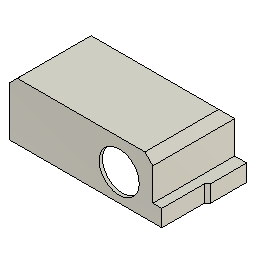
1_Assembly Camera v20 (Autodesk Fusion 360 archive; units mm, degrees)
design "Camera"
Autodesk Fusion 360 part; units mm, degrees
sketch "Cam" plane through (0, 0, 0) normal (0, 0, 1) x (1, 0, 0)
  line L0 (-62.75, 35.75) -> (62.75, 35.75)
  line L1 (62.75, 35.75) -> (62.75, -35.75)
  line L2 (62.75, -35.75) -> (-62.75, -35.75)
  line L3 (-62.75, -35.75) -> (-62.75, 35.75)
  line L4 (62.75, -35.75) -> (70.55, -35.75)
  line L5 (70.55, -35.75) -> (70.55, 1.75)
  line L6 (70.55, 1.75) -> (73.25, 4.45)
  line L7 (73.25, 4.45) -> (73.25, 35.75)
  line L8 (73.25, 35.75) -> (62.75, 35.75)
  line L9 (-62.75, 35.75) -> (62.75, -35.75) construction
  line L10 (-62.75, -35.75) -> (62.75, 35.75) construction
  dimension "d122" = 125.5
  dimension "d123" = 71.5
  dimension "d126" = 10.5
  dimension "d127" = 7.8
  dimension "d395" = 135
  dimension "d396" = 31.3
  constraint horizontal L0
  constraint vertical L1
  constraint horizontal L2
  constraint vertical L3
  constraint perpendicular L1 L4
  constraint perpendicular L4 L5
  constraint perpendicular L4 L7
  constraint perpendicular L7 L8
  constraint coincident origin L10
  constraint coincident origin L9
  measures "d122" distance of L0.start L0.end
  measures "d123" distance of L0.start L2.end
  measures "d126" distance of L0.end L7.end
  measures "d127" distance of L1.end L4.end
  measures "d395" angle of L5 L6
  measures "d396" distance of L6.end L7.end
extrude "Extrude2" add sketch "Cam" along normal blind 50 contours L0 L1 L2 L3
chamfer "Chamfer2" distance 7 angle 45 3 edges at (-62.75, 0, 50) (0, 35.75, 50) (62.75, 0, 50)
shell "Shell1" thickness 3 removed faces 1 at (20.9167, -11.9167, 0)
extrude "Extrude3" add sketch "Cam" along normal blind 14.7 contours L1 L4 L5 L6 L7 L8
sketch "Cam hole" plane through (0, -35.75, 0) normal (0, -1, 0) x (1, 0, 0)
  line L0 (62.75, 43) -> (55.75, 50)
  line L1 (55.75, 50) -> (-55.75, 50)
  line L2 (-55.75, 50) -> (-62.75, 43)
  line L3 (-62.75, 43) -> (-62.75, 0)
  line L4 (-62.75, 0) -> (70.55, 0)
  line L5 (70.55, 0) -> (70.55, 14.7)
  line L6 (70.55, 14.7) -> (62.75, 14.7)
  line L7 (62.75, 14.7) -> (62.75, 43)
  circle A0 centre (33.25, 23.5) radius 17.5
  dimension "d137" = 35
  dimension "d154" = 23.5
  dimension "d155" = 29.5
  measures "d137" diameter of A0
  measures "d154" distance of L4 A0.centre
  measures "d155" distance of L7 A0.centre
extrude "Extrude4" cut sketch "Cam hole" against normal blind 20 contours A0
sketch "Cam Fix" plane through (0, 0, 0) normal (0, 0, -1) x (1, 0, 0)
  line L0 (-59.75, -32.75) -> (-59.75, 32.75)
  line L1 (-59.75, 32.75) -> (59.75, 32.75)
  line L2 (59.75, 32.75) -> (59.75, -32.75)
  line L3 (59.75, -32.75) -> (-59.75, -32.75)
  line L4 (70.55, 35.75) -> (-62.75, 35.75)
  line L5 (-62.75, 35.75) -> (-62.75, -35.75)
  line L6 (-62.75, -35.75) -> (73.25, -35.75)
  line L7 (73.25, -35.75) -> (73.25, -4.45)
  line L8 (73.25, -4.45) -> (70.55, -1.75)
  line L9 (70.55, -1.75) -> (70.55, 35.75)
  line L10 (-59.75, 32.75) -> (-49.75, 32.75)
  line L11 (-49.75, 32.75) -> (-49.75, 22.75)
  line L12 (-49.75, 22.75) -> (-59.75, 22.75)
  line L13 (-59.75, 22.75) -> (-59.75, 32.75)
  line L14 (-59.75, -32.75) -> (-49.75, -32.75)
  line L15 (-49.75, -32.75) -> (-49.75, -22.75)
  line L16 (-49.75, -22.75) -> (-59.75, -22.75)
  line L17 (-59.75, -22.75) -> (-59.75, -32.75)
  line L18 (-59.75, 32.75) -> (-49.75, 22.75) construction
  line L19 (-59.75, -22.75) -> (-49.75, -32.75) construction
  circle A0 centre (-54.75, 27.75) radius 2.6
  circle A1 centre (64.75, 27.75) radius 2.6
  circle A2 centre (64.75, -27.75) radius 2.6
  circle A3 centre (-54.75, -27.75) radius 2.6
  line L20 (59.75, 32.75) -> (69.75, 32.75)
  line L21 (69.75, 32.75) -> (69.75, 22.75)
  line L22 (69.75, 22.75) -> (59.75, 22.75)
  line L23 (59.75, 22.75) -> (59.75, 32.75)
  line L24 (59.75, -22.75) -> (69.75, -22.75)
  line L25 (69.75, -22.75) -> (69.75, -32.75)
  line L26 (69.75, -32.75) -> (59.75, -32.75)
  line L27 (59.75, -32.75) -> (59.75, -22.75)
  line L28 (59.75, -22.75) -> (69.75, -32.75) construction
  line L29 (59.75, 32.75) -> (69.75, 22.75) construction
  dimension "d140" = 10
  dimension "d141" = 10
  dimension "d142" = 10
  dimension "d143" = 10
  dimension "d148" = 5.2
  dimension "d149" = 5.2
  dimension "d150" = 5.2
  dimension "d151" = 5.2
  dimension "d156" = 10
  dimension "d157" = 10
  dimension "d158" = 10
  dimension "d159" = 10
  constraint horizontal L10
  constraint vertical L11
  constraint horizontal L12
  constraint vertical L13
  constraint coincident L0.end L1.start
  constraint horizontal L14
  constraint vertical L15
  constraint horizontal L16
  constraint vertical L17
  constraint coincident L0.start L3.end
  constraint coincident L1.end L2.start
  constraint midpoint L18 A0.centre
  constraint midpoint L19 A3.centre
  constraint horizontal L20
  constraint vertical L21
  constraint horizontal L22
  constraint vertical L23
  constraint horizontal L24
  constraint vertical L25
  constraint horizontal L26
  constraint vertical L27
  constraint midpoint A1.centre L29
  constraint midpoint A2.centre L28
  constraint coincident L2.end L3.start
  measures "d140" distance of L0.end L10.end
  measures "d141" distance of L0.end L12.end
  measures "d142" distance of L0.start L14.end
  measures "d143" distance of L0.start L16.end
  measures "d148" diameter of A0
  measures "d149" diameter of A1
  measures "d150" diameter of A2
  measures "d151" diameter of A3
  measures "d156" distance of L1.end L20.end
  measures "d157" distance of L1.end L22.end
  measures "d158" distance of L24.start L24.end
  measures "d159" distance of L2.end L24.start
extrude "Extrude5" add sketch "Cam Fix" against normal blind 10 contours L0 L3 L14 L15 L16 L17 | L0 L1 L10 L11 L12 L13 | A0 | A3
extrude "Extrude6" cut sketch "Cam Fix" against normal blind 3.1 contours A0 | A1 | A2 | A3
equation "Trous_Vis_diam2 = 2.2 mm"
equation "d175 = Trous_Vis_diam2"
equation "d176 = Trous_Vis_diam2"
equation "d179 = Trous_Vis_diam2"
equation "d180 = Trous_Vis_diam2"
equation "d183 = Trous_Vis_diam2"
equation "d185 = Trous_Vis_diam2"
equation "d186 = Trous_Vis_diam2"
equation "d187 = Trous_Vis_diam2"
equation "d198 = Trous_Vis_diam2"
equation "d199 = Trous_Vis_diam2"
equation "d200 = Trous_Vis_diam2"
equation "d201 = Trous_Vis_diam2"
equation "d365 = Trous_Vis_diam2"
equation "d367 = Trous_Vis_diam2"
equation "d368 = Trous_Vis_diam2"
equation "d369 = Trous_Vis_diam2"
named bodies: "Cam"

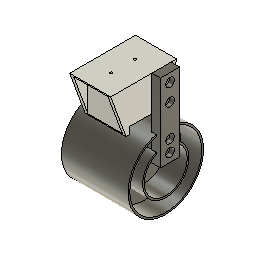
design "Under Camera"
Autodesk Fusion 360 part; units mm, degrees
sketch "Sketch1" plane through (0, -227.1998, 566.5) normal (1, 0, 0) x (0, 1, 0) in component "Under Cam"
  line L0 (-26, -3.5) -> (12.5005, -3.5)
  line L1 (12.5005, -3.5) -> (8.0001, -24)
  line L2 (8.0001, -24) -> (-15.3, -24)
  line L3 (-15.3, -24) -> (-15.3, -28.1777)
  line L4 (-15.3, -28.1777) -> (-17, -28.1777)
  line L5 (-17, -28.1777) -> (-26, -3.5)
  line L6 (3.7005, -3.5) -> (3.7005, -24) construction
  circle A0 centre (3.7005, -8.5) radius 0.75
  circle A1 centre (3.7005, -18.5) radius 0.75
  dimension "d282" = 8.8
  dimension "d283" = 1.5
  dimension "d284" = 5
  dimension "d285" = 1.5
  dimension "d286" = 10
  constraint horizontal L0
  constraint parallel L0 L2
  constraint perpendicular L2 L3
  constraint perpendicular L3 L4
  constraint coincident L0 L6.start
  constraint coincident L2 L6.end
  constraint perpendicular L2 L6
  constraint coincident L6 A0.centre
  constraint coincident L6 A1.centre
  measures "d282" distance of L0.end L6.start
  measures "d283" diameter of A0
  measures "d284" distance of L0 A0.centre
  measures "d285" diameter of A1
  measures "d286" distance of A0.centre A1.centre
extrude "Extrude1" add sketch "Sketch1" against normal blind 24 contours L0 L1 L2 L3 L4 L5 | A0 | A1 makes body 1 in component "Under Cam"
ref_plane "WorkPlane2" through (-12, -257.4998, 540.4111) normal (0, 1, 0) x (0, 0, -1) in component "Under Cam"
sketch "Sketch2" plane through (-71.456, -257.4998, 540.4111) normal (0, 1, 0) x (1, 0, 0) in component "Under Cam"
  line L0 (71.456, 2.0889) -> (71.456, -22.5888)
  line L1 (71.456, -22.5888) -> (47.456, -22.5888)
  line L2 (47.456, -22.5888) -> (47.456, 2.0889)
  line L3 (47.456, 2.0889) -> (71.456, 2.0889)
  line L4 (49.456, -21.5888) -> (69.456, -21.5888)
  line L5 (69.456, -21.5888) -> (69.456, 2.0889)
  line L6 (69.456, 2.0889) -> (49.456, 2.0889)
  line L7 (49.456, 2.0889) -> (49.456, -21.5888)
  dimension "d273" = 2
  dimension "d274" = 2
  dimension "d275" = 1
  constraint horizontal L4
  constraint vertical L5
  constraint horizontal L6
  constraint vertical L7
  constraint coincident L3 L5.end
  measures "d273" horizontal distance of L1.end L4.start
  measures "d274" horizontal distance of L0.end L4.end
  measures "d275" vertical distance of L0.end L4.end
extrude "Extrude2" cut sketch "Sketch2" along normal blind 13 contours L3 L4 L5 L6 L7 bodies 1 in component "Under Cam"
extrude "Extrude4" cut sketch "Sketch1" against normal blind 10 contours A0 | A1 bodies 1 in component "Under Cam"
sketch "Sketch3" plane through (0, -227.1998, 566.5) normal (1, 0, 0) x (0, 1, 0) in component "Under Cam"
  line L0 (-1.8995, -3.5) -> (9.3005, -3.5)
  line L1 (9.3005, -3.5) -> (9.3005, -49)
  line L2 (9.3005, -49) -> (-1.8995, -49)
  line L3 (-1.8995, -49) -> (-1.8995, -3.5)
  line L4 (-26, -3.5) -> (12.5005, -3.5)
  line L5 (-26, -3.5) -> (12.5005, -3.5) construction
  line L6 (3.7005, -3.5) -> (3.7005, -49) construction
  circle A0 centre (3.7005, -8.5) radius 1.1
  circle A1 centre (3.7005, -18.5) radius 1.1
  line L7 (3.7005, -49) -> (3.7005, -77.9127) construction
  point P0 (3.7005, -8.5)
  point P1 (3.7005, -18.5)
  dimension "d278" = 11.2
  dimension "d281" = 8.8
  dimension "d289" = 2.2
  dimension "d290" = 2.2
  constraint horizontal L0
  constraint vertical L1
  constraint horizontal L2
  constraint vertical L3
  constraint coincident L4.start L5.start
  constraint coincident L4.end L5.end
  constraint coincident L0.end L5
  constraint midpoint L0 L6.start
  constraint perpendicular L0 L6
  constraint coincident P0 A0.centre
  constraint coincident P1 A1.centre
  constraint perpendicular L2 L7
  measures "d278" distance of L0.start L0.end
  measures "d281" distance of L4.end L6.start
  measures "d289" diameter of A0
  measures "d290" diameter of A1
extrude "Extrude3" add sketch "Sketch3" along normal blind 5 separate body makes body 2 in component "Under Cam"
sketch "Sketch4" plane through (5, 0, 0) normal (1, 0, 0) x (0, 1, 0) in component "Under Cam"
  circle A0 centre (-223.4993, 548) radius 1.1
  circle A1 centre (-223.4993, 558) radius 1.1
  line L0 (-229.0993, 517.5) -> (-217.8993, 517.5)
  line L1 (-217.8993, 517.5) -> (-217.8993, 563)
  line L2 (-217.8993, 563) -> (-229.0993, 563)
  line L3 (-229.0993, 563) -> (-229.0993, 517.5)
  circle A2 centre (-223.4993, 558) radius 2.5
  circle A3 centre (-223.4993, 548) radius 2.5
  line L4 (-223.4993, 548) -> (-223.4993, 517.5) construction
  dimension "d291" = 5
  dimension "d292" = 5
  constraint concentric A1 A2
  constraint concentric A0 A3
  constraint coincident A0.centre A3.centre
  constraint midpoint L0 L4.end
  measures "d291" diameter of A2
  measures "d292" diameter of A3
sketch "Sketch6" plane through (0, -227.1998, 566.5) normal (1, 0, 0) x (0, 1, 0) in component "Under Cam"
  line L0 (-1.8995, -49) -> (9.3005, -49)
  line L1 (3.7005, -49) -> (3.7005, -32.5726) construction
  circle A0 centre (3.7005, -54.5726) radius 22
  circle A1 centre (3.7005, -54.5726) radius 21
  circle A2 centre (3.7005, -54.5726) radius 13.5
  circle A3 centre (3.7005, -54.5726) radius 12.5
  line L2 (9.3005, -49) -> (9.3005, -33.2972)
  line L3 (-1.8995, -49) -> (-1.8995, -33.2972)
  circle A4 centre (3.7005, -37) radius 0.75
  circle A5 centre (3.7005, -44) radius 0.75
  point P0 (9.3005, -49)
  point P1 (-1.8995, -49)
  dimension "d295" = 44
  dimension "d298" = -1
  dimension "d299" = -8.5
  dimension "d300" = -9.5
  dimension "d305" = 1.5
  dimension "d306" = 1.5
  dimension "d307" = 5
  dimension "d308" = 7
  constraint coincident P1 L0.start
  constraint coincident P0 L0.end
  constraint midpoint L0 L1.start
  constraint perpendicular L0 L1
  constraint coincident L1 A0.centre
  constraint coincident A0 L2.end
  constraint vertical L2
  constraint coincident A0 L3.end
  constraint perpendicular L0 L3
  constraint coincident L1.end A0
  constraint coincident L1 A4.centre
  constraint coincident L1 A5.centre
  measures "d295" diameter of A0
  measures "d305" diameter of A4
  measures "d306" diameter of A5
  measures "d307" distance of L1.start A5.centre
  measures "d308" distance of A4.centre A5.centre
extrude "Extrude6" add sketch "Sketch6" against normal blind 36.5 separate body contours L0 A3 L2 L3 | L0 A3 L2 L3 | A2 A3 L2 L3 | A2 A3 L2 L3 | A1 A2 L2 L3 | A1 A2 L2 L3 | A0 A1 L2 L3 | A0 A1 L2 L3 | A4 | A5 makes body 3 in component "Under Cam"
extrude "Extrude7" cut sketch "Sketch6" against normal blind 10 contours L0 A3 L2 L3 | A1 A2 L2 L3 picked at (3.532, -55.0208) picked at (-4.7622, -38.1727) bodies 3 in component "Under Cam"
extrude "Extrude8" add sketch "Sketch6" along normal blind 2.5 contours A2 A3 L2 L3 | A0 A1 L2 L3 picked at (-3.0056, -43.6595) picked at (-3.9032, -34.6912) bodies 3 in component "Under Cam"
extrude "Extrude9" cut sketch "Sketch6" against normal blind 10 contours A4 | A5 bodies 3 in component "Under Cam"
sketch "Sketch7" plane through (5, 0, 0) normal (1, 0, 0) x (0, 1, 0) in component "Under Cam"
  line L0 (-229.0993, 517.5) -> (-217.8993, 517.5)
  line L1 (-217.8993, 517.5) -> (-217.8993, 563)
  line L2 (-217.8993, 563) -> (-229.0993, 563)
  line L3 (-229.0993, 563) -> (-229.0993, 517.5)
  circle A0 centre (-223.4993, 529.5) radius 1.1
  circle A1 centre (-223.4993, 522.5) radius 1.1
  circle A2 centre (-223.4993, 529.5) radius 2.5
  circle A3 centre (-223.4993, 522.5) radius 2.5
  circle A4 centre (-223.4993, 558) radius 1.1
  circle A5 centre (-223.4993, 548) radius 1.1
  point P0 (-223.4993, 529.5)
  point P1 (-223.4993, 522.5)
  dimension "d311" = 2.2
  dimension "d312" = 2.2
  dimension "d313" = 5
  dimension "d314" = 5
  constraint coincident P0 A0.centre
  constraint coincident P1 A1.centre
  constraint concentric A0 A2
  constraint concentric A1 A3
  measures "d311" diameter of A0
  measures "d312" diameter of A1
  measures "d313" diameter of A2
  measures "d314" diameter of A3
extrude "Extrude5" cut sketch "Sketch4" sketch "Sketch7" against normal blind 2.5 contours A2 | A3 of sketch 2 contours A2 | A3 bodies 2 in component "Under Cam"
extrude "Extrude10" cut sketch "Sketch7" against normal blind 5 contours A0 | A1 bodies 2 in component "Under Cam"
sketch "Sketch8" plane through (0, 0, 563) normal (0, 0, 1) x (-1, 0, 0) in component "Under Cam"
  line L0 (0, 253.1998) -> (0, 214.6993)
  line L1 (0, 214.6993) -> (24, 214.6993)
  line L2 (24, 214.6993) -> (24, 253.1998)
  line L3 (24, 253.1998) -> (0, 253.1998)
  line L4 (12, 214.6993) -> (12, 253.1998) construction
  circle A0 centre (12, 226.9495) radius 0.75
  circle A1 centre (12, 240.9495) radius 0.75
  line L5 (12, 233.9495) -> (0, 233.9495) construction
  dimension "d389" = 1.5
  dimension "d390" = 1.5
  dimension "d391" = 7
  dimension "d392" = 7
  constraint midpoint L1 L4.start
  constraint midpoint L3 L4.end
  constraint coincident L4 A0.centre
  constraint coincident L4 A1.centre
  constraint midpoint L4 L5.start
  constraint midpoint L0 L5.end
  measures "d389" diameter of A0
  measures "d390" diameter of A1
  measures "d391" distance of A1.centre L5.start
  measures "d392" distance of A0.centre L5.start
extrude "Extrude11" cut sketch "Sketch8" against normal blind 10 contours A0 | A1 bodies 1 in component "Under Cam"
component "Under Cam" placed x (1, 0, 0) y (0, 1, 0) z (0, 0, 1) at (0, 0, 0)
equation "Trous_Vis_diam2 = 2.2 mm"
equation "d175 = Trous_Vis_diam2"
equation "d176 = Trous_Vis_diam2"
equation "d179 = Trous_Vis_diam2"
equation "d180 = Trous_Vis_diam2"
equation "d183 = Trous_Vis_diam2"
equation "d185 = Trous_Vis_diam2"
equation "d186 = Trous_Vis_diam2"
equation "d187 = Trous_Vis_diam2"
equation "d198 = Trous_Vis_diam2"
equation "d199 = Trous_Vis_diam2"
equation "d200 = Trous_Vis_diam2"
equation "d201 = Trous_Vis_diam2"
equation "d365 = Trous_Vis_diam2"
equation "d367 = Trous_Vis_diam2"
equation "d368 = Trous_Vis_diam2"
equation "d369 = Trous_Vis_diam2"
named bodies: "support double cam", "fixation latérale", "Cylindre"

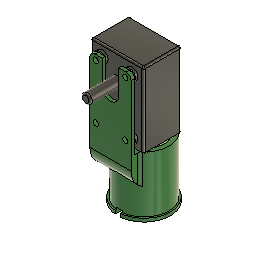
design "Support motor rotor"
Autodesk Fusion 360 part; units mm, degrees
sketch "Sketch1" plane through (0, 0, 0) normal (0, 0, 1) x (1, 0, 0)
  circle A0 centre (0, 0) radius 12.4
  circle A1 centre (0, 0) radius 13.4
  circle A2 centre (0, 0) radius 1.1
  circle A3 centre (0, 0) radius 15
  circle A4 centre (0, 0) radius 16
  dimension "d1" = 24.8
  dimension "d2" = 1
  dimension "d8" = 2.2
  dimension "d103" = 30
  dimension "d117" = 32
  constraint coincident A0.centre A1.centre
  constraint concentric A0 A2
  measures "d1" diameter of A0
  measures "d8" diameter of A2
  measures "d103" diameter of A3
  measures "d117" diameter of A4
extrude "Extrude1" add sketch "Sketch1" against normal blind 2 contours A0 | A1 | A3 makes body 1
extrude "Extrude2" add sketch "Sketch1" along normal blind 34 contours A1 bodies 1
ref_plane "WorkPlane2" through (0, -15, 0) normal (0, 1, 0) x (0, 0, 1)
sketch "Sketch3" plane through (0, -15, 0) normal (0, 1, 0) x (1, 0, 0)
sketch "Sketch4" plane through (0, -15, 0) normal (0, 1, 0) x (1, 0, 0)
  line L0 (-13.4, -34) -> (13.4, -34)
  line L1 (-8.4, -34) -> (-3.3, -34)
  line L2 (7.8, -34) -> (7.8, -14)
  line L3 (7.8, -14) -> (-8.4, -14)
  line L4 (-8.4, -14) -> (-8.4, -34)
  line L5 (9.2, -77) -> (9.2, -34)
  line L6 (9.2, -34) -> (-15.8, -34)
  line L7 (-15.8, -34) -> (-15.8, -77)
  line L8 (-3.3, -77) -> (-3.3, -34) construction
  line L9 (-8.3, -77) -> (-8.3, -62.0106)
  line L10 (1.7, -77) -> (1.7, -62.0106)
  line L11 (-15.8, -77) -> (-8.3, -77)
  line L12 (1.7, -77) -> (9.2, -77)
  arc A0 (1.7, -62.0106) -> (-8.3, -62.0106) centre (-3.3, -62.0106) ccw
  line L13 (-12.3, -74) -> (5.7, -74) construction
  line L14 (5.7, -74) -> (5.7, -41) construction
  line L15 (5.7, -41) -> (-12.3, -41) construction
  line L16 (-12.3, -41) -> (-12.3, -74) construction
  circle A1 centre (5.7, -41) radius 1.6
  circle A2 centre (-12.3, -41) radius 1.6
  circle A3 centre (-12.3, -74) radius 1.6
  circle A4 centre (5.7, -74) radius 1.6
  line L17 (13.4, 0) -> (-13.4, 0)
  line L18 (9.2, -34) -> (-15.8, -34)
  line L19 (-15.8, -34) -> (-15.8, -14)
  line L20 (-15.8, -14) -> (9.2, -14)
  line L21 (9.2, -14) -> (9.2, -34)
  dimension "d55" = 5
  dimension "d57" = 25
  dimension "d58" = 43
  dimension "d62" = 7.4
  dimension "d64" = 10
  dimension "d66" = 33
  dimension "d67" = 18
  dimension "d69" = 3.5
  dimension "d70" = 3.5
  dimension "d71" = 3.2
  dimension "d72" = 3.2
  dimension "d73" = 3.2
  dimension "d74" = 3.2
  dimension "d76" = 7
  dimension "d85" = 20
  constraint horizontal L1
  constraint vertical L2
  constraint horizontal L3
  constraint vertical L4
  constraint coincident L0 L1.start
  constraint horizontal L11
  constraint vertical L5
  constraint horizontal L6
  constraint vertical L7
  constraint coincident L1.start L6
  constraint midpoint L6 L1.end
  constraint coincident L8 A0.centre
  constraint tangent L9 A0
  constraint perpendicular L9 L11
  constraint coincident L10.start L11
  constraint tangent L10 A0
  constraint perpendicular L10 L11
  constraint collinear L11 L12
  constraint coincident L8.start L11
  constraint horizontal L13
  constraint vertical L14
  constraint horizontal L15
  constraint vertical L16
  constraint coincident L14.end L15.start
  constraint coincident L15.end L16.start
  constraint coincident L13.start L16.end
  constraint coincident L13.end L14.start
  constraint horizontal L18
  constraint vertical L19
  constraint horizontal L20
  constraint vertical L21
  constraint coincident L6.end L7.start
  measures "d55" distance of L0.start L1.start
  measures "d57" distance of L7.end L5.start
  measures "d58" distance of L7.end L6.end
  measures "d62" distance of L1.start L6.end
  measures "d64" diameter of A0
  measures "d66" distance of L13.start L15.end
  measures "d67" distance of L13.start L13.end
  measures "d69" distance of L5 L14.end
  measures "d70" distance of L7 L15.end
  measures "d71" diameter of A1
  measures "d72" diameter of A2
  measures "d73" diameter of A3
  measures "d74" diameter of A4
  measures "d76" distance of L1 L14.end
  measures "d85" distance of L2.start L2.end
extrude "Extrude6" add sketch "Sketch4" against normal blind 2 separate body makes body 2
extrude "Extrude7" add sketch "Sketch4" along normal blind 13 contours L0 L4 L6 L18 L19 L20 | L0 L1 L2 L3 L4 L6 L18 L20 | L0 L2 L6 L18 L20 L21 bodies 1 2
extrude "Extrude9" cut 1 faces at (8.5831, -0.6707, 0) along direction (0, 0, 1) blind 35 on bodies 1 bodies 1
extrude "Extrude10" add 1 faces at (14.4108, -0.7452, 0) along direction (0, 0, 1) blind 34 on bodies 1 bodies 1
fillet "Fillet3" radius 3 2 edges at (9.2, -16, 77) (-15.8, -16, 77) on bodies 1
fillet "Fillet2" radius 12.5 1 edges at (-3.3, -17, 14) on bodies 1
fillet "Fillet6" radius 2.5 1 edges at (9.2, -11.8474, 25.1937) on bodies 1
extrude "Extrude13" add sketch "Sketch1" against normal blind 2 contours A4 bodies 1
sketch "Sketch6" plane through (0, 0, -2) normal (0, 0, -1) x (1, 0, 0)
  line L0 (1.6, -16.8286) -> (-1.6, -16.8286)
  line L1 (-1.6, -16.8286) -> (-1.6, 16.8286)
  line L2 (-1.6, 16.8286) -> (1.6, 16.8286)
  line L3 (1.6, 16.8286) -> (1.6, -16.8286)
  line L4 (1.6, -16.8286) -> (-1.6, 16.8286) construction
  line L5 (-1.6, -16.8286) -> (1.6, 16.8286) construction
  circle A0 centre (0, 0) radius 7.5
  circle A1 centre (0, 0) radius 1.1
  circle A2 centre (0, 0) radius 16
  dimension "d108" = 3.2
  dimension "d111" = 15
  constraint perpendicular L0 L1
  constraint parallel L0 L2
  constraint parallel L1 L3
  constraint horizontal L0
  constraint coincident L4 A0.centre
  constraint coincident L5 A0.centre
  constraint coincident A0.centre A1.centre
  measures "d108" distance of L1.end L2.end
  measures "d111" diameter of A0
extrude "Extrude11" cut sketch "Sketch6" against normal blind 3 contours L1 L3 A0 A2 | L1 L3 A0 A2 bodies 1
fillet "Fillet7" radius 5 1 edges at (-15.8, -2, 24) on bodies 1
sketch "Sketch7" plane through (0, 0, -2) normal (0, 0, -1) x (1, 0, 0)
  circle A0 centre (0, 0) radius 12.4
  line L0 (0, 0) -> (0, -12.4) construction
  line L1 (-10.745, 10.3072) -> (-12.3181, 8.3641)
  arc A1 (-12.3181, 8.3641) -> (-8.802, 8.7342) centre (-10.375, 6.7911) ccw
  arc A2 (-10.375, 6.7911) -> (-10.745, 10.3072) centre (-8.802, 8.7342) ccw
  dimension "d115" = 5
  dimension "d116" = 5
  constraint coincident A0.centre L0.start
  constraint coincident A0 L0.end
  constraint vertical L0
  constraint coincident A0 A1.centre
  constraint coincident A0 A1.end
  constraint tangent L1 A1
  measures "d115" diameter of A1
  measures "d116" diameter of A2
extrude "Extrude12" cut sketch "Sketch7" against normal through all contours A0 L1 A1 A2 bodies 1
copy_body "Body->Comp2" bodies 1 removing the originals makes body 3 in component "Support Motor"
sketch "Sketch1 (2)" plane through (0, 0, 0) normal (0, 0, 1) x (1, 0, 0) in component "Head Motor v3"
  line L0 (-16, -23) -> (16, -23)
  line L1 (16, -23) -> (16, 23)
  line L2 (16, 23) -> (-16, 23)
  line L3 (-16, 23) -> (-16, -23)
  line L4 (-16, -23) -> (16, 23) construction
  line L5 (16, -23) -> (-16, 23) construction
  dimension "d1_1" = 46
  dimension "d2_1" = 32
  constraint perpendicular L0 L1
  constraint parallel L0 L2
  constraint parallel L1 L3
  constraint horizontal L0
  constraint coincident L4 origin
  constraint coincident L5 origin
  measures "d1_1" distance of L0.end L1.end
  measures "d2_1" distance of L1.end L2.end
extrude "Extrude1'" add sketch "Sketch1 (2)" along normal blind 23 separate body makes body 4 in component "Head Motor v3"
sketch "Sketch2" plane through (0, 0, 23) normal (0, 0, 1) x (-1, 0, 0) in component "Head Motor v3"
  line L0 (16, -23) -> (16, 23)
  line L1 (16, 23) -> (-16, 23)
  line L2 (-16, 23) -> (-16, -23)
  line L3 (-16, -23) -> (16, -23)
  line L4 (-9, 16.5) -> (9, 16.5) construction
  line L5 (9, 16.5) -> (9, -16.5) construction
  line L6 (9, -16.5) -> (-9, -16.5) construction
  line L7 (-9, -16.5) -> (-9, 16.5) construction
  line L8 (-9, 16.5) -> (9, -16.5) construction
  line L9 (9, 16.5) -> (-9, -16.5) construction
  circle A0 centre (-9, -16.5) radius 3.5
  circle A1 centre (9, -16.5) radius 3.5
  circle A2 centre (-9, 16.5) radius 3.5
  circle A3 centre (9, 16.5) radius 3.5
  line L10 (0, -23) -> (0, 23) construction
  circle A4 centre (0, -8) radius 3
  circle A5 centre (9, -16.5) radius 1.5
  circle A6 centre (-9, -16.5) radius 1.5
  circle A7 centre (9, 16.5) radius 1.5
  circle A8 centre (-9, 16.5) radius 1.5
  dimension "d5_1" = 33
  dimension "d6_1" = 18
  dimension "d7" = 7
  dimension "d8_1" = 7
  dimension "d9" = 7
  dimension "d10" = 7
  dimension "d13" = 6
  dimension "d14" = 15
  dimension "d34" = 3
  dimension "d35" = 3
  dimension "d36" = 3
  dimension "d37" = 3
  constraint perpendicular L4 L5
  constraint parallel L4 L6
  constraint parallel L5 L7
  constraint horizontal L4
  constraint coincident L8 origin
  constraint coincident L9 origin
  constraint coincident L6.end L7.start
  constraint coincident L5.end L6.start
  constraint coincident L4.start L7.end
  constraint coincident L4.end L5.start
  constraint midpoint L3 L10.start
  constraint midpoint L1 L10.end
  constraint coincident L10 A4.centre
  constraint concentric A1 A5
  constraint concentric A3 A7
  constraint concentric A2 A8
  measures "d5_1" distance of L4.end L5.end
  measures "d6_1" distance of L5.end L6.end
  measures "d7" diameter of A0
  measures "d8_1" diameter of A1
  measures "d9" diameter of A2
  measures "d10" diameter of A3
  measures "d13" diameter of A4
  measures "d14" distance of L3 A4.centre
  measures "d34" diameter of A5
  measures "d35" diameter of A6
  measures "d36" diameter of A7
  measures "d37" diameter of A8
extrude "Extrude2'" add sketch "Sketch2" along normal blind 2 contours A0 | A1 | A2 | A3 bodies 4 in component "Head Motor v3"
extrude "Extrude3" add sketch "Sketch2" along normal blind 19 contours A4 bodies 4 in component "Head Motor v3"
fillet "Fillet1" radius 1 4 faces at (16, -7.6667, 7.6667) (-5.3333, -23, 7.6667) (-16, 7.6667, 7.6667) (5.3333, 23, 7.6667) on bodies 4 in component "Head Motor v3"
fillet "Fillet2'" radius 0.5 1 edges at (-5.7369, -15.2343, 25) 4 faces at (6.1853, 16.7484, 25) (6.1853, -16.2516, 25) (-11.8147, 16.7484, 25) (-11.8147, -16.2516, 25) on bodies 4 in component "Head Motor v3"
fillet "Fillet3'" radius 1 1 faces at (0.5, 8.866, 42) on bodies 4 in component "Head Motor v3"
sketch "Sketch4 (2)" plane through (-3, 23, 11.5) normal (0, 1, 0) x (-1, 0, 0) in component "Head Motor v3"
sketch "Sketch5" plane through (0, -23, 0) normal (0, -1, 0) x (1, 0, 0) in component "Head Motor v3"
  line L0 (-15, 1) -> (15, 1)
  line L1 (15, 1) -> (15, 22)
  line L2 (15, 22) -> (-15, 22)
  line L3 (-15, 22) -> (-15, 1)
  circle A0 centre (3, 10) radius 12
  point P0 (16, 22)
  dimension "d25" = 24
  dimension "d26" = 10
  dimension "d27" = 13
  measures "d25" diameter of A0
  measures "d26" vertical distance of origin A0.centre
  measures "d27" horizontal distance of A0.centre P0
extrude "Extrude5" add sketch "Sketch5" along normal blind 31 contours L0 A0 | L0 A0 bodies 4 in component "Head Motor v3"
sketch "Sketch8" plane through (0, -54, 0) normal (0, -1, 0) x (1, 0, 0) in component "Head Motor v3"
  circle A0 centre (3, 10) radius 12
  circle A1 centre (3, 10) radius 11.8
  dimension "d31" = -0.2
extrude "Extrude6'" cut sketch "Sketch8" against normal blind 1 contours A1 bodies 4 in component "Head Motor v3"
component "Support Motor" placed x (1, 0, 0) y (0, 1, 0) z (0, 0, 1) at (0, 0, 0)
component "Head Motor v3" placed x (1, 0, 0) y (0, 0, 1) z (0, -1, 0) at (-3.3, 10, 57.5)
named bodies: "Support Motor"

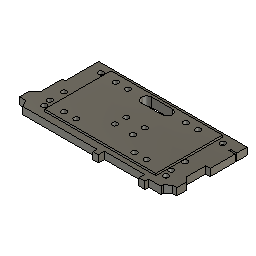
design "Support Camera"
Autodesk Fusion 360 part; units mm, degrees
sketch "Support Cam" plane through (0, 0, 0) normal (0, 0, 1) x (1, 0, 0)
  line L0 (-198.7446, -257.0866) -> (-125.8054, -257.0866)
  line L1 (-125.8054, -257.0866) -> (-125.8054, -260.9951)
  line L2 (-125.8054, -260.9951) -> (-120.4545, -260.9951)
  line L3 (-120.4545, -260.9951) -> (-120.4545, -255.1026)
  line L4 (-120.4545, -255.1026) -> (-80.9396, -255.1026)
  line L5 (-80.9396, -255.1026) -> (-80.9396, -260.7322)
  line L6 (-80.9396, -260.7322) -> (-75.0474, -260.7322)
  line L7 (-75.0474, -260.7322) -> (-75.0474, -257.0778)
  line L8 (-75.0474, -257.0778) -> (-62.9514, -257.0778)
  line L9 (-62.9514, -257.0778) -> (-62.9514, -254.5567)
  line L10 (-62.9514, -254.5567) -> (-58.1923, -250.6191)
  line L11 (-58.1923, -250.6191) -> (-53.9714, -250.6191)
  line L12 (-53.9714, -250.6191) -> (-53.9714, -241.0645)
  line L13 (-53.9714, -241.0645) -> (-58.456, -236.613)
  line L14 (-58.456, -236.613) -> (-58.456, -217.7866)
  line L15 (-58.456, -217.7866) -> (-53.9714, -217.7866)
  line L16 (-53.9714, -217.7866) -> (-53.9714, -193.3927)
  line L17 (-53.9714, -193.3927) -> (-60.1213, -193.3927)
  line L18 (-60.1213, -193.3927) -> (-60.1213, -191.7009)
  line L19 (-60.1213, -191.7009) -> (-53.9714, -191.7009)
  line L20 (-53.9714, -191.7009) -> (-53.9714, -181.6027)
  line L21 (-53.9714, -181.6027) -> (-199.5171, -181.6027)
  line L22 (-199.5171, -181.6027) -> (-199.5171, -214.5082)
  line L23 (-199.5171, -214.5082) -> (-202.4466, -214.5082)
  line L24 (-202.4466, -214.5082) -> (-202.4466, -235.0144)
  line L25 (-202.4466, -235.0144) -> (-208.3055, -241.7413)
  line L26 (-208.3055, -241.7413) -> (-208.3055, -250.4212)
  line L27 (-208.3055, -250.4212) -> (-202.4466, -250.4212)
  line L28 (-202.4466, -250.4212) -> (-198.7446, -257.0866)
  line L29 (-202.4466, -214.5082) -> (-178.9466, -214.5082) construction
  line L30 (-178.9466, -214.5082) -> (-178.9466, -253.5082) construction
  line L31 (-178.9466, -253.5082) -> (-202.4466, -253.5082) construction
  line L32 (-202.4466, -253.5082) -> (-202.4466, -214.5082) construction
  line L33 (-83.4128, -214.476) -> (-59.9128, -214.476) construction
  line L34 (-59.9128, -214.476) -> (-59.9128, -253.476) construction
  line L35 (-59.9128, -253.476) -> (-83.4128, -253.476) construction
  line L36 (-83.4128, -253.476) -> (-83.4128, -214.476) construction
  line L37 (-176.7676, -200.3683) -> (-154.7676, -200.3683) construction
  line L38 (-154.7676, -200.3683) -> (-154.7676, -185.3683) construction
  line L39 (-154.7676, -185.3683) -> (-176.7676, -185.3683) construction
  line L40 (-176.7676, -185.3683) -> (-176.7676, -200.3683) construction
  line L41 (-107.7676, -185.3683) -> (-107.7676, -200.3683) construction
  line L42 (-107.7676, -200.3683) -> (-85.7676, -200.3683) construction
  line L43 (-85.7676, -200.3683) -> (-85.7676, -185.3683) construction
  line L44 (-85.7676, -185.3683) -> (-107.7676, -185.3683) construction
  line L45 (-190.6966, -253.5082) -> (-190.6966, -214.5082) construction
  circle A0 centre (-190.6966, -238.5082) radius 1.1
  circle A1 centre (-190.6966, -224.5082) radius 1.1
  line L46 (-71.6628, -253.476) -> (-71.6628, -214.476) construction
  circle A2 centre (-71.6628, -238.476) radius 1.1
  circle A3 centre (-71.6628, -224.476) radius 1.1
  line L47 (-176.7676, -192.8683) -> (-154.7676, -192.8683) construction
  line L48 (-107.7676, -192.8683) -> (-85.7676, -192.8683) construction
  circle A4 centre (-171.7676, -192.8683) radius 1.1
  circle A5 centre (-159.7676, -192.8683) radius 1.1
  circle A6 centre (-102.7676, -192.8683) radius 1.1
  circle A7 centre (-90.7676, -192.8683) radius 1.1
  line L49 (-141.6035, -233.9087) -> (-141.6035, -212.4087) construction
  line L50 (-141.6035, -212.4087) -> (-113.6035, -212.4087) construction
  line L51 (-113.6035, -212.4087) -> (-113.6035, -233.9087) construction
  line L52 (-113.6035, -233.9087) -> (-141.6035, -233.9087) construction
  line L53 (-118.6035, -228.9087) -> (-136.6035, -228.9087) construction
  line L54 (-136.6035, -228.9087) -> (-136.6035, -217.4087) construction
  line L55 (-136.6035, -217.4087) -> (-118.6035, -217.4087) construction
  line L56 (-118.6035, -217.4087) -> (-118.6035, -228.9087) construction
  circle A8 centre (-136.6035, -228.9087) radius 1.1
  circle A9 centre (-118.6035, -228.9087) radius 1.1
  circle A10 centre (-118.6035, -217.4087) radius 1.1
  circle A11 centre (-136.6035, -217.4087) radius 1.1
  circle A12 centre (-188.7259, -245.8252) radius 2.6
  circle A13 centre (-188.7259, -190.3252) radius 2.6
  circle A14 centre (-69.2259, -190.3252) radius 2.6
  circle A15 centre (-69.2259, -245.8252) radius 2.6
  line L57 (-154.7676, -192.8683) -> (-107.7676, -192.8683) construction
  line L58 (-141.2676, -197.8683) -> (-121.2676, -197.8683)
  arc A16 (-121.2676, -197.8683) -> (-121.2676, -187.8683) centre (-121.2676, -192.8683) ccw
  line L59 (-121.2676, -187.8683) -> (-141.2676, -187.8683)
  arc A17 (-141.2676, -187.8683) -> (-141.2676, -197.8683) centre (-141.2676, -192.8683) ccw
  line L60 (-141.2676, -192.8683) -> (-121.2676, -192.8683) construction
  line L61 (-183.7259, -250.8252) -> (-74.2259, -250.8252) construction
  line L62 (-74.2259, -250.8252) -> (-74.2259, -185.3252) construction
  line L63 (-74.2259, -185.3252) -> (-183.7259, -185.3252) construction
  line L64 (-183.7259, -185.3252) -> (-183.7259, -250.8252) construction
  line L65 (-183.5759, -185.4752) -> (-183.5759, -250.6752)
  line L66 (-183.5759, -250.6752) -> (-74.3759, -250.6752)
  line L67 (-74.3759, -250.6752) -> (-74.3759, -185.4752)
  line L68 (-74.3759, -185.4752) -> (-183.5759, -185.4752)
  circle A18 centre (-136.6035, -217.4087) radius 2.5
  circle A19 centre (-118.6035, -217.4087) radius 2.5
  circle A20 centre (-136.6035, -228.9087) radius 2.5
  circle A21 centre (-118.6035, -228.9087) radius 2.5
  circle A22 centre (-71.6628, -224.476) radius 2.5
  circle A23 centre (-71.6628, -238.476) radius 2.5
  circle A24 centre (-190.6966, -224.5082) radius 2.5
  circle A25 centre (-190.6966, -238.5082) radius 2.5
  circle A26 centre (-171.7676, -192.8683) radius 2.5
  circle A27 centre (-159.7676, -192.8683) radius 2.5
  circle A28 centre (-102.7676, -192.8683) radius 2.5
  circle A29 centre (-90.7676, -192.8683) radius 2.5
  line L69 (-176.7676, -243.3252) -> (-154.7676, -243.3252) construction
  circle A30 centre (-171.7676, -243.3252) radius 1.1
  circle A31 centre (-159.7676, -243.3252) radius 1.1
  circle A32 centre (-171.7676, -243.3252) radius 2.5
  circle A33 centre (-159.7676, -243.3252) radius 2.5
  circle A34 centre (-90.7676, -243.3252) radius 2.5
  circle A35 centre (-102.7676, -243.3252) radius 2.5
  circle A36 centre (-90.7676, -243.3252) radius 1.1
  line L70 (-107.7676, -243.3252) -> (-85.7676, -243.3252) construction
  circle A37 centre (-102.7676, -243.3252) radius 1.1
  point P0 (-188.7259, -245.8252)
  point P1 (-188.7259, -190.3252)
  point P2 (-69.2259, -190.3252)
  point P3 (-69.2259, -245.8252)
  point P4 (-131.2676, -192.8683)
  point P5 (-183.7259, -185.3252)
  point P6 (-183.7259, -250.8252)
  point P7 (-74.2259, -250.8252)
  point P8 (-74.2259, -185.3252)
  dimension "d165" = 23.5
  dimension "d166" = 39
  dimension "d167" = 23.5
  dimension "d168" = 39
  dimension "d169" = 22
  dimension "d170" = 15
  dimension "d171" = 22
  dimension "d172" = 15
  dimension "d175" = 2.2
  dimension "d176" = 2.2
  dimension "d177" = 10
  dimension "d178" = 15
  dimension "d179" = 2.2
  dimension "d180" = 2.2
  dimension "d181" = 10
  dimension "d182" = 15
  dimension "d183" = 2.2
  dimension "d184" = 5
  dimension "d185" = 2.2
  dimension "d186" = 2.2
  dimension "d187" = 2.2
  dimension "d188" = 5
  dimension "d189" = 5
  dimension "d190" = 5
  dimension "d195" = 21.5
  dimension "d196" = 28
  dimension "d197" = 5
  dimension "d198" = 2.2
  dimension "d199" = 2.2
  dimension "d200" = 2.2
  dimension "d201" = 2.2
  dimension "d204" = 5.2
  dimension "d205" = 5.2
  dimension "d206" = 5.2
  dimension "d207" = 5.2
  dimension "d210" = 10
  dimension "d248" = -0.15
  dimension "d253" = 5
  dimension "d254" = 5
  dimension "d255" = 5
  dimension "d256" = 5
  dimension "d259" = 5
  dimension "d260" = 5
  dimension "d261" = 5
  dimension "d262" = 5
  dimension "d265" = 5
  dimension "d266" = 5
  dimension "d267" = 5
  dimension "d268" = 5
  dimension "d365" = 2.2
  dimension "d366" = 5
  dimension "d367" = 2.2
  dimension "d368" = 2.2
  dimension "d369" = 2.2
  dimension "d370" = 5
  dimension "d371" = 5
  dimension "d372" = 5
  dimension "d373" = 5
  dimension "d374" = 5
  dimension "d375" = 5
  dimension "d376" = 5
  dimension "d377" = 7.5
  dimension "d378" = 7.5
  constraint horizontal L0
  constraint perpendicular L0 L1
  constraint perpendicular L1 L2
  constraint perpendicular L2 L3
  constraint perpendicular L3 L4
  constraint perpendicular L4 L5
  constraint perpendicular L3 L6
  constraint perpendicular L6 L7
  constraint perpendicular L7 L8
  constraint perpendicular L8 L9
  constraint perpendicular L9 L11
  constraint perpendicular L11 L12
  constraint perpendicular L11 L14
  constraint perpendicular L14 L15
  constraint perpendicular L15 L16
  constraint perpendicular L16 L17
  constraint perpendicular L17 L18
  constraint perpendicular L18 L19
  constraint perpendicular L19 L20
  constraint perpendicular L3 L21
  constraint perpendicular L21 L22
  constraint perpendicular L22 L23
  constraint perpendicular L23 L24
  constraint parallel L24 L26
  constraint perpendicular L26 L27
  constraint horizontal L29
  constraint vertical L30
  constraint horizontal L31
  constraint vertical L32
  constraint horizontal L33
  constraint vertical L34
  constraint horizontal L35
  constraint vertical L36
  constraint horizontal L37
  constraint vertical L38
  constraint horizontal L39
  constraint vertical L40
  constraint horizontal L42
  constraint vertical L43
  constraint horizontal L44
  constraint vertical L41
  constraint midpoint L31 L45.start
  constraint midpoint L29 L45.end
  constraint coincident L45 A0.centre
  constraint coincident L45 A1.centre
  constraint midpoint L35 L46.start
  constraint midpoint L33 L46.end
  constraint coincident L46 A2.centre
  constraint coincident L46 A3.centre
  constraint midpoint L40 L47.start
  constraint midpoint L38 L47.end
  constraint midpoint L41 L48.start
  constraint midpoint L43 L48.end
  constraint coincident L47 A4.centre
  constraint coincident L47 A5.centre
  constraint coincident L48 A6.centre
  constraint coincident L48 A7.centre
  constraint vertical L49
  constraint perpendicular L49 L50
  constraint perpendicular L50 L51
  constraint perpendicular L51 L52
  constraint coincident L53.end L54.start
  constraint coincident L53.start L56.end
  constraint coincident L55.end L56.start
  constraint coincident L54.end L55.start
  constraint coincident P0 A12.centre
  constraint coincident P1 A13.centre
  constraint coincident P2 A14.centre
  constraint coincident P3 A15.centre
  constraint perpendicular L41 L57
  constraint tangent L58 A16
  constraint tangent A16 L59
  constraint parallel L58 L59
  constraint tangent L59 A17
  constraint tangent L58 A17
  constraint perpendicular L30 L60
  constraint midpoint L57 P4
  constraint midpoint L60 P4
  constraint horizontal L61
  constraint vertical L62
  constraint horizontal L63
  constraint vertical L64
  constraint coincident P8 L62.end
  constraint coincident P6 L61.start
  constraint concentric A11 A18
  constraint concentric A10 A19
  constraint concentric A8 A20
  constraint concentric A9 A21
  constraint concentric A3 A22
  constraint concentric A2 A23
  constraint concentric A1 A24
  constraint concentric A0 A25
  constraint concentric A4 A26
  constraint concentric A5 A27
  constraint concentric A6 A28
  constraint concentric A7 A29
  constraint coincident A30.centre L69
  constraint coincident A31.centre L69
  constraint coincident A35.centre L70
  constraint coincident A34.centre L70
  constraint concentric A30 A32
  constraint concentric A31 A33
  constraint concentric A35 A37
  constraint concentric A34 A36
  measures "d165" distance of L23.end L29.end
  measures "d166" distance of L23.end L31.end
  measures "d167" distance of L33.start L33.end
  measures "d168" distance of L33.start L35.end
  measures "d169" distance of L37.start L37.end
  measures "d170" distance of L37.start L39.end
  measures "d171" distance of L42.end L41.end
  measures "d172" distance of L41.start L41.end
  measures "d175" diameter of A0
  measures "d176" diameter of A1
  measures "d177" distance of L45.end A1.centre
  measures "d178" distance of L31 A0.centre
  measures "d179" diameter of A2
  measures "d180" diameter of A3
  measures "d181" distance of L46.end A3.centre
  measures "d182" distance of L46.start A2.centre
  measures "d183" diameter of A4
  measures "d184" distance of L47.start A4.centre
  measures "d185" diameter of A5
  measures "d186" diameter of A6
  measures "d187" diameter of A7
  measures "d188" distance of L48.start A6.centre
  measures "d189" distance of L48.end A7.centre
  measures "d190" distance of L47.end A5.centre
  measures "d195" distance of L49.start L49.end
  measures "d196" distance of L49.start L51.end
  measures "d198" diameter of A8
  measures "d199" diameter of A9
  measures "d200" diameter of A10
  measures "d201" diameter of A11
  measures "d204" diameter of A12
  measures "d205" diameter of A13
  measures "d206" diameter of A14
  measures "d207" diameter of A15
  measures "d210" diameter of A16
  measures "d253" diameter of A18
  measures "d254" diameter of A19
  measures "d255" diameter of A20
  measures "d256" diameter of A21
  measures "d259" diameter of A22
  measures "d260" diameter of A23
  measures "d261" diameter of A24
  measures "d262" diameter of A25
  measures "d265" diameter of A26
  measures "d266" diameter of A27
  measures "d267" diameter of A28
  measures "d268" diameter of A29
  measures "d365" diameter of A30
  measures "d366" distance of A30.centre L69.start
  measures "d367" diameter of A31
  measures "d368" diameter of A37
  measures "d369" diameter of A36
  measures "d370" distance of A35.centre L70.start
  measures "d371" distance of L70.end A34.centre
  measures "d372" distance of L69.end A31.centre
  measures "d373" diameter of A32
  measures "d374" diameter of A33
  measures "d375" diameter of A35
  measures "d376" diameter of A34
  measures "d377" distance of L61 L70.start
  measures "d378" distance of L61 L69.end
extrude "Extrude9" add sketch "Support Cam" against normal blind 7 contours L0 L1 L2 L3 L4 L5 L6 L7 L8 L9 L10 L11 L12 L13 L14 L15 L16 L17 L18 L19 L20 L21 L22 L23 L24 L25 L26 L27 L28 | A12 | A13 | A14 | A15 | L65 L66 L67 L68 | A18 | A19 | A20 | A21 | A22 | A23 | A24 | A25 | A26 | A27 | A28 | A29 | A32 | A33 | A34 | A35
extrude "Extrude15" add sketch "Support Cam" along normal blind 2 contours L65 L66 L67 L68
extrude "Extrude16" cut sketch "Support Cam" against normal blind 3.1 contours A12 | A13 | A14 | A15
extrude "Extrude18" cut sketch "Support Cam" against normal blind 3.5 contours A18 | A19 | A20 | A21 | A22 | A23 | A24 | A25 | A26 | A27 | A28 | A29 | A32 | A33 | A34 | A35
equation "d175 = Trous_Vis_diam2"
equation "d176 = Trous_Vis_diam2"
equation "d179 = Trous_Vis_diam2"
equation "d180 = Trous_Vis_diam2"
equation "d183 = Trous_Vis_diam2"
equation "d185 = Trous_Vis_diam2"
equation "d186 = Trous_Vis_diam2"
equation "d187 = Trous_Vis_diam2"
equation "d198 = Trous_Vis_diam2"
equation "d199 = Trous_Vis_diam2"
equation "d200 = Trous_Vis_diam2"
equation "d201 = Trous_Vis_diam2"
equation "d365 = Trous_Vis_diam2"
equation "d367 = Trous_Vis_diam2"
equation "d368 = Trous_Vis_diam2"
equation "d369 = Trous_Vis_diam2"
equation "Trous_Vis_diam2 = 2.2 mm"
equation "Χ = "
equation "Φ = "
equation "Υ = "
equation "Τ = "
equation "Σ = "
equation "Ψ = "
equation "Ͳ = "
equation "³ = "
equation "µ = "
equation "ӿ = "
equation "ԅ = "
named bodies: "Support Cam"
